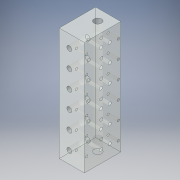
# Autodesk Inventor part: SX10_manifold6
Saved by Autodesk Inventor 2019 (Build 230136000, 136)
## iProperties
Created: 2018-12-18
Part Number: SX10_manifold6
Material: Generic
Document SubType Name: Modeling
Designer: Brian
Density: 1 g/cm^3
Appearance: Default
Author: Brian
Autodesk Inventor part; units mm, degrees
ref_plane "YZ Plane" through (0, 0, 0) normal (1, 0, 0) x (0, 1, 0)
ref_plane "XZ Plane" through (0, 0, 0) normal (0, 1, 0) x (-1, 0, 0)
ref_plane "XY Plane" through (0, 0, 0) normal (0, 0, 1) x (1, 0, 0)
sketch "Sketch1" plane through (0, 0, 0) normal (0, 1, 0) x (-1, 0, 0)
  line L0 (0, 0) -> (-31.75, 0)
  line L1 (-31.75, 0) -> (-31.75, -46)
  line L2 (-31.75, -46) -> (0, -46)
  line L3 (0, -46) -> (0, 0)
  dimension "d0" = 31.75
  dimension "d1" = 46
  constraints: 8 end point, 2 parallel, 1 horizontal, 1 perpendicular
  measures "d0" distance of L2.end L1.end
  measures "d1" distance of L1.end L0.end
extrude "Extrusion1" add sketch "Sketch1" along normal blind 143.002
sketch "Sketch3" plane through (31.75, 0, 0) normal (1, 0, 0) x (0, 0, -1)
  line L0 (0, 143.002) -> (46, 143.002) projected
  line L1 (46, 0) -> (46, 143.002) projected
  line L2 (46, 0) -> (46, 143.002) projected
  point P0 (0, 0)
  point P1 (21, 15.2412)
  point P2 (32, 37.5932)
  point P3 (32, 59.9452)
  point P4 (21, 37.5932)
  point P5 (21, 59.9452)
  point P6 (32, 82.2972)
  point P7 (32.2323, 104.648)
  point P8 (21, 82.2972)
  point P9 (21.2323, 104.648)
  point P10 (32, 127)
  point P11 (32, 15.2412)
  dimension "d18" = 16.002
  dimension "d19" = 22.352
  dimension "d20" = 22.352
  dimension "d21" = 22.352
  dimension "d22" = 22.352
  dimension "d31" = 22.352
  dimension "d32" = 14
  dimension "d33" = 14
  dimension "d34" = 14
  dimension "d35" = 14
  dimension "d36" = 14
  dimension "d37" = 11
  dimension "d38" = 11
  dimension "d39" = 11
  dimension "d40" = 11
  dimension "d42" = 11
  dimension "d172" = 22.352
  dimension "d173" = 22.3508
  dimension "d174" = 22.352
  dimension "d175" = 22.352
  dimension "d176" = 22.352
  measures "d18" distance from line of L0 point (32, 127)
  measures "d19" vertical distance of point (32, 127) point (32.232, 104.648)
  measures "d20" distance of point (32.232, 104.648) point (32, 82.297)
  measures "d21" distance of point (32, 82.297) point (32, 59.945)
  measures "d22" distance of point (32, 59.945) point (32, 37.593)
  measures "d31" distance of point (32, 37.593) point (32, 15.241)
  measures "d32" distance from line of L1 point (32, 127)
  measures "d33" distance from line of point (32, 82.297) L2
  measures "d34" distance from line of L1 point (32, 59.945)
  measures "d35" distance from line of L1 point (32, 37.593)
  measures "d36" distance from line of L1 point (32, 15.241)
  measures "d37" distance of point (32.232, 104.648) point (21.232, 104.648)
  measures "d38" distance of point (32, 82.297) point (21, 82.297)
  measures "d39" distance of point (32, 59.945) point (21, 59.945)
  measures "d40" distance of point (32, 37.593) point (21, 37.593)
  measures "d42" distance of point (32, 15.241) point (21, 15.241)
  measures "d172" vertical distance of point (32, 127) point (21.232, 104.648)
  measures "d173" vertical distance of point (21.232, 104.648) point (21, 82.297)
  measures "d174" distance of point (21, 82.297) point (21, 59.945)
  measures "d175" distance of point (21, 59.945) point (21, 37.593)
  measures "d176" distance of point (21, 37.593) point (21, 15.241)
hole "Hole2" at (31.75, 15.2412, -21) at (31.75, 37.5932, -32) at (31.75, 59.9452, -32) at (31.75, 37.5932, -21) at (31.75, 59.9452, -21) at (31.75, 82.2972, -32) at (31.75, 104.648, -32.2323) at (31.75, 82.2972, -21) at (31.75, 104.648, -21.2323) at (31.75, 127, -32) direction (-1, 0, 0) diameter 4 depth 17 tip angle 118
sketch "Sketch5" plane through (31.75, 0, 0) normal (1, 0, 0) x (0, 0, -1)
  line L0 (46, 0) -> (46, 143.002) projected
  line L1 (0, 0) -> (46, 0) projected
  line L2 (0, 143.002) -> (46, 143.002) projected
  point P0 (32, 16.002)
  point P1 (21, 127)
  dimension "d50" = 14
  dimension "d51" = 16.002
  dimension "d52" = 16.002
  dimension "d53" = 25
  measures "d50" distance from line of L0 point (32, 16.002)
  measures "d51" distance from line of L1 point (32, 16.002)
  measures "d52" distance from line of L2 point (21, 127)
  measures "d53" distance from line of L0 point (21, 127)
hole "Hole4" at (31.75, 16.002, -32) at (31.75, 127, -21) direction (-1, 0, 0) diameter 4 depth 17 tip angle 118
sketch "Sketch6" plane through (31.75, 0, 0) normal (1, 0, 0) x (0, 0, -1)
  line L0 (0, 143.002) -> (46, 143.002) projected
  line L1 (46, 0) -> (46, 143.002) projected
  line L2 (0, 0) -> (0, 143.002) projected
  point P0 (43, 13.742)
  point P1 (43, 36.094)
  point P2 (43, 58.446)
  point P3 (43, 80.798)
  point P4 (43, 103.15)
  point P5 (43, 125.502)
  point P6 (3, 16.742)
  point P7 (3, 39.094)
  point P8 (3, 61.446)
  point P9 (3, 83.798)
  point P10 (3, 106.15)
  point P11 (3, 128.502)
  dimension "d61" = 17.5
  dimension "d62" = 14.5
  dimension "d63" = 3
  dimension "d64" = 22.352
  dimension "d65" = 3
  dimension "d66" = 22.352
  dimension "d67" = 3
  dimension "d68" = 22.352
  dimension "d69" = 3
  dimension "d70" = 22.352
  dimension "d71" = 3
  dimension "d72" = 22.352
  dimension "d73" = 3
  dimension "d75" = 22.352
  dimension "d77" = 22.352
  dimension "d79" = 22.352
  dimension "d81" = 22.352
  dimension "d83" = 22.352
  dimension "d85" = 40
  dimension "d86" = 40
  dimension "d87" = 40
  dimension "d88" = 40
  dimension "d89" = 40
  dimension "d90" = 40
  measures "d61" distance from line of L0 point (43, 125.502)
  measures "d62" distance from line of L0 point (3, 128.502)
  measures "d63" distance from line of L1 point (43, 125.502)
  measures "d64" distance of point (43, 125.502) point (43, 103.15)
  measures "d65" distance from line of L1 point (43, 103.15)
  measures "d66" distance of point (43, 103.15) point (43, 80.798)
  measures "d67" distance from line of L1 point (43, 80.798)
  measures "d68" distance of point (43, 80.798) point (43, 58.446)
  measures "d69" distance from line of L1 point (43, 58.446)
  measures "d70" distance of point (43, 58.446) point (43, 36.094)
  measures "d71" distance from line of L1 point (43, 36.094)
  measures "d72" distance of point (43, 36.094) point (43, 13.742)
  measures "d73" distance from line of L1 point (43, 13.742)
  measures "d75" distance of point (3, 128.502) point (3, 106.15)
  measures "d77" distance of point (3, 106.15) point (3, 83.798)
  measures "d79" distance of point (3, 83.798) point (3, 61.446)
  measures "d81" distance of point (3, 61.446) point (3, 39.094)
  measures "d83" distance of point (3, 39.094) point (3, 16.742)
  measures "d85" horizontal distance of point (43, 125.502) point (3, 128.502)
  measures "d86" horizontal distance of point (43, 103.15) point (3, 106.15)
  measures "d87" horizontal distance of point (43, 80.798) point (3, 83.798)
  measures "d88" horizontal distance of point (43, 58.446) point (3, 61.446)
  measures "d89" horizontal distance of point (43, 36.094) point (3, 39.094)
  measures "d90" horizontal distance of point (43, 13.742) point (3, 16.742)
hole "Hole5" at (31.75, 13.742, -43) at (31.75, 36.094, -43) at (31.75, 58.446, -43) at (31.75, 80.798, -43) at (31.75, 103.15, -43) at (31.75, 125.502, -43) at (31.75, 16.742, -3) at (31.75, 39.094, -3) at (31.75, 61.446, -3) at (31.75, 83.798, -3) at (31.75, 106.15, -3) at (31.75, 128.502, -3) direction (-1, 0, 0) diameter 3 depth 13 tip angle 118
thread "Thread1" size "M3x0.5" class "6H" standard "ANSI Metric M Profile" full length
thread "Thread2" size "5-40 UNC" class "2B" standard "ANSI Unified Screw Threads" full length
thread "Thread3" size "5-40 UNC" class "2B" standard "ANSI Unified Screw Threads" full length
thread "Thread4" size "5-40 UNC" class "2B" standard "ANSI Unified Screw Threads" full length
thread "Thread5" size "5-40 UNC" class "2B" standard "ANSI Unified Screw Threads" full length
thread "Thread6" size "M3x0.5" class "6H" standard "ANSI Metric M Profile" full length
thread "Thread7" size "M3x0.5" class "6H" standard "ANSI Metric M Profile" full length
thread "Thread8" size "M3x0.5" class "6H" standard "ANSI Metric M Profile" full length
thread "Thread9" size "M3x0.5" class "6H" standard "ANSI Metric M Profile" full length
thread "Thread10" size "M3x0.5" class "6H" standard "ANSI Metric M Profile" full length
thread "Thread11" size "M3x0.5" class "6H" standard "ANSI Metric M Profile" full length
thread "Thread12" size "M3x0.5" class "6H" standard "ANSI Metric M Profile" full length
thread "Thread13" size "M3x0.5" class "6H" standard "ANSI Metric M Profile" full length
thread "Thread14" size "M3x0.5" class "6H" standard "ANSI Metric M Profile" full length
thread "Thread15" size "M3x0.5" class "6H" standard "ANSI Metric M Profile" full length
thread "Thread16" size "M3x0.5" class "6H" standard "ANSI Metric M Profile" full length
thread "Thread17" size "M3x0.5" class "6H" standard "ANSI Metric M Profile" full length
thread "Thread18" size "M3x0.5" class "6H" standard "ANSI Metric M Profile" full length
sketch "Sketch7" plane through (0, 0, 0) normal (0, -1, 0) x (1, 0, 0)
  line L0 (31.75, -46) -> (0, -46) projected
  line L1 (31.75, 0) -> (31.75, -46) projected
  point P0 (0, 0)
  point P1 (16.75, -32)
  dimension "d136" = 14
  dimension "d137" = 15
  measures "d136" distance from line of L0 point (16.75, -32)
  measures "d137" distance from line of L1 point (16.75, -32)
hole "Hole6" at (16.75, 0, -32) direction (0, 1, 0) diameter 9.525 depth 152.4 tip angle 118
thread "Thread19" size "3/8" designation "3/8 - 18 NPT" standard "NPT" length 15.2654
sketch "Sketch8" plane through (0, 0, 0) normal (0, 0, 1) x (1, 0, 0)
  line L0 (31.75, 0) -> (31.75, 143.002) projected
  line L1 (0, 0) -> (31.75, 0) projected
  line L2 (0, 143.002) -> (31.75, 143.002) projected
  point P0 (12.75, 15.24)
  point P1 (12.75, 37.592)
  point P2 (12.75, 59.944)
  point P3 (12.75, 82.296)
  point P4 (12.75, 104.648)
  point P5 (12.75, 127)
  dimension "d145" = 19
  dimension "d147" = 22.352
  dimension "d148" = 22.352
  dimension "d149" = 22.352
  dimension "d150" = 22.352
  dimension "d151" = 22.352
  dimension "d152" = 19
  dimension "d153" = 19
  dimension "d154" = 19
  dimension "d155" = 19
  dimension "d156" = 19
  dimension "d171" = 16.002
  measures "d145" distance from line of L0 point (12.75, 15.24)
  measures "d147" distance of point (12.75, 15.24) point (12.75, 37.592)
  measures "d148" distance of point (12.75, 37.592) point (12.75, 59.944)
  measures "d149" distance of point (12.75, 59.944) point (12.75, 82.296)
  measures "d150" distance of point (12.75, 82.296) point (12.75, 104.648)
  measures "d151" distance of point (12.75, 104.648) point (12.75, 127)
  measures "d152" distance from line of L0 point (12.75, 37.592)
  measures "d153" distance from line of L0 point (12.75, 59.944)
  measures "d154" distance from line of L0 point (12.75, 82.296)
  measures "d155" distance from line of L0 point (12.75, 104.648)
  measures "d156" distance from line of L0 point (12.75, 127)
  measures "d171" distance from line of L2 point (12.75, 127)
hole "Hole7" at (12.75, 15.24, 0) at (12.75, 37.592, 0) at (12.75, 59.944, 0) at (12.75, 82.296, 0) at (12.75, 104.648, 0) at (12.75, 127, 0) direction (0, 0, -1) diameter 6.35 depth 23.25
thread "Thread20" size "1/4" designation "1/4 - 18 NPT" standard "NPT" length 15.113
thread "Thread21" size "1/4" designation "1/4 - 18 NPT" standard "NPT" length 15.113
thread "Thread22" size "1/4" designation "1/4 - 18 NPT" standard "NPT" length 15.113
thread "Thread23" size "1/4" designation "1/4 - 18 NPT" standard "NPT" length 15.113
thread "Thread24" size "1/4" designation "1/4 - 18 NPT" standard "NPT" length 15.113
thread "Thread25" size "1/4" designation "1/4 - 18 NPT" standard "NPT" length 15.113
thread "Thread26" size "3/8" designation "3/8 - 18 NPT" standard "NPT" length 15.2654
body "Solid1"
